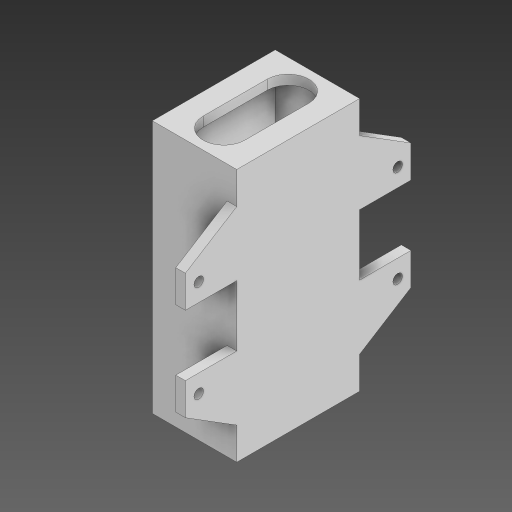
# Autodesk Inventor part: akb_mount
Saved by Autodesk Inventor 2023 (Build 270158000, 158)
## iProperties
Created: 2025-07-15
Part Number: akb_mount
Material: Типовые
Document SubType Name: Modeling
Designer: daa
Density: 1 g/cm^3
Appearance: По умолчанию
Author: daa
Autodesk Inventor part; units mm, degrees
ref_plane "YZ Plane" through (0, 0, 0) normal (1, 0, 0) x (0, 1, 0)
ref_plane "XZ Plane" through (0, 0, 0) normal (0, 1, 0) x (-1, 0, 0)
ref_plane "XY Plane" through (0, 0, 0) normal (0, 0, 1) x (1, 0, 0)
sketch "Эскиз1" plane through (0, 0, 0) normal (0, 1, 0) x (-1, 0, 0)
  line L0 (11, 17) -> (-11, 17)
  line L1 (-11, 17) -> (-11, -17)
  line L2 (-11, -17) -> (11, -17)
  line L3 (11, -17) -> (11, 17)
  line L4 (11, 17) -> (-11, -17) construction
  line L5 (11.65, 17.65) -> (-11.65, 17.65)
  line L6 (-11.65, 17.65) -> (-11.65, -17.65)
  line L7 (-11.65, -17.65) -> (11.65, -17.65)
  line L8 (11.65, -17.65) -> (11.65, 17.65)
  line L9 (11.65, 17.65) -> (-11.65, -17.65) construction
  line L10 (13.15, 19.15) -> (-13.15, 19.15)
  line L11 (-13.15, 19.15) -> (-13.15, -19.15)
  line L12 (-13.15, -19.15) -> (13.15, -19.15)
  line L13 (13.15, -19.15) -> (13.15, 19.15)
  line L14 (13.15, 19.15) -> (-13.15, -19.15) construction
  point P0 (0, 0)
  point P1 (0, 0)
  point P2 (0, 0)
  dimension "d0" = 22
  dimension "d1" = 34
  dimension "d2" = 23.3
  dimension "d3" = 35.3
  dimension "d4" = 26.3
  dimension "d5" = 38.3
  constraints: 30 end point, 6 parallel, 3 horizontal, 3 midpoint, 3 perpendicular, 1 coincident
  measures "d0" distance of L2.end L2.start
  measures "d1" distance of L2.start L0.end
  measures "d2" distance of L7.start L7.end
  measures "d3" distance of L7.end L5.start
  measures "d4" distance of L12.start L12.end
  measures "d5" distance of L10.end L12.start
extrude "Выдавливание1" add sketch "Эскиз1" along normal blind 76 contours L13 L12 L11 L10
sketch "Эскиз2" plane through (0, 76, 0) normal (0, 1, 0) x (1, 0, 0)
  line L0 (11, 17) -> (-11, 17)
  line L1 (-11, 17) -> (-11, -17)
  line L2 (-11, -17) -> (11, -17)
  line L3 (11, -17) -> (11, 17)
  line L4 (11, 17) -> (-11, -17) construction
  line L5 (11.65, 17.65) -> (-11.65, 17.65)
  line L6 (-11.65, 17.65) -> (-11.65, -17.65)
  line L7 (-11.65, -17.65) -> (11.65, -17.65)
  line L8 (11.65, -17.65) -> (11.65, 17.65)
  line L9 (11.65, 17.65) -> (-11.65, -17.65) construction
  line L10 (13.15, 19.15) -> (-13.15, 19.15)
  line L11 (-13.15, 19.15) -> (-13.15, -19.15)
  line L12 (-13.15, -19.15) -> (13.15, -19.15)
  line L13 (13.15, -19.15) -> (13.15, 19.15)
  line L14 (13.15, 19.15) -> (-13.15, -19.15) construction
  point P0 (0, 0)
  point P1 (0, 0)
  point P2 (0, 0)
  dimension "d10" = 22
  dimension "d11" = 34
  dimension "d12" = 23.3
  dimension "d13" = 35.3
  dimension "d14" = 26.3
  dimension "d15" = 38.3
  constraints: 30 end point, 6 parallel, 3 horizontal, 3 midpoint, 3 perpendicular, 1 coincident
  measures "d10" distance of L2.end L2.start
  measures "d11" distance of L2.start L0.end
  measures "d12" distance of L7.start L7.end
  measures "d13" distance of L7.end L5.start
  measures "d14" distance of L12.start L12.end
  measures "d15" distance of L10.end L12.start
extrude "Выдавливание2" add sketch "Эскиз2" along normal blind 3 contours L3 L2 L1 L0 | L8 L7 L6 L5 | L13 L12 L11 L10
sketch "Эскиз3" plane through (0, 79, 0) normal (0, 1, 0) x (1, 0, 0)
  line L0 (0, 10) -> (0, -10) construction
  line L1 (-6.5, 10) -> (-6.5, -10)
  line L2 (6.5, -10) -> (6.5, 10)
  arc A0 (6.5, 10) -> (-6.5, 10) centre (0, 10) ccw
  arc A1 (-6.5, -10) -> (6.5, -10) centre (0, -10) ccw
  line L3 (13.15, -19.15) -> (13.15, 19.15) projected
  line L4 (13.15, 19.15) -> (-13.15, 19.15) projected
  point P0 (0, 0)
  point P1 (13.15, 0)
  dimension "d21" = 20
  dimension "d22" = 13
  dimension "d23" = 6.65
  dimension "d24" = 19.15
  constraints: 8 end point, 4 point on circle, 4 tangent, 2 centre point, 2 midpoint, 1 parallel, 1 vertical
  measures "d21" distance of L0.start L0.end
  measures "d22" diameter of A1
  measures "d23" distance from line of point (13.15, 0) L2
  measures "d24" distance from line of L4 point (0, 0)
extrude "Выдавливание3" cut sketch "Эскиз3" against normal blind 3
sketch "Эскиз4" plane through (13.15, 0, 19.15) normal (1, 0, 0) x (0, 0, -1)
  line L0 (0, 0) -> (0, 79) projected
  line L1 (38.3, 0) -> (38.3, 79) projected
  line L2 (0, 79) -> (38.3, 79)
  line L3 (38.3, 79) -> (38.3, 0)
  line L4 (38.3, 0) -> (0, 0)
  line L5 (0, 0) -> (0, 79)
  circle A0 centre (50.15, 54.6) radius 1.5
  line L6 (50.15, 54.6) -> (-11.85, 54.6)
  line L7 (-11.85, 54.6) -> (-11.85, 24.4)
  line L8 (-11.85, 24.4) -> (50.15, 24.4)
  line L9 (50.15, 24.4) -> (50.15, 54.6)
  circle A1 centre (-11.85, 54.6) radius 1.5
  circle A2 centre (-11.85, 24.4) radius 1.5
  circle A3 centre (50.15, 24.4) radius 1.5
  line L10 (38.3, 79) -> (0, 79) projected
  line L11 (19.15, 79) -> (19.15, 0)
  line L12 (0, 39.5) -> (38.3, 39.5)
  line L13 (38.3, 39.5) -> (0, 39.5)
  circle A4 centre (-11.85, 24.4) radius 1.5
  line L14 (38.3, 49) -> (54.3, 49)
  line L15 (54.3, 49) -> (54.3, 59)
  line L16 (54.3, 59) -> (38.3, 69)
  line L17 (38.3, 30) -> (54.3, 30)
  line L18 (54.3, 30) -> (54.3, 20)
  line L19 (54.3, 20) -> (38.3, 10)
  line L20 (-16, 20) -> (0, 10)
  line L21 (-16, 30) -> (-16, 20)
  line L22 (0, 30) -> (-16, 30)
  line L23 (0, 49) -> (-16, 49)
  line L24 (-16, 49) -> (-16, 59)
  line L25 (-16, 59) -> (0, 69)
  point P0 (54.3, 54)
  point P1 (54.3, 25)
  point P2 (50.15, 30)
  point P3 (50.15, 49)
  point P4 (-11.85, 49)
  point P5 (-11.85, 30)
  dimension "d50" = 3
  dimension "d53" = 62
  dimension "d54" = 30.2
  dimension "d55" = 11.85
  dimension "d56" = 3
  dimension "d57" = 3
  dimension "d61" = 24.4
  dimension "d62" = 30
  dimension "d63" = 10
  dimension "d64" = 10
  dimension "d65" = 4.15
  constraints: 46 end point, 16 symmetric about line, 5 centre point, 5 midpoint, 4 parallel, 3 coincident, 3 horizontal, 2 perpendicular, 2 point on line, 1 vertical, 1 other
  measures "d50" diameter of A0
  measures "d53" distance of L8.end L7.end
  measures "d54" distance of L7.end L6.end
  measures "d55" distance between parallel lines of L0 L7
  measures "d56" diameter of A1
  measures "d57" diameter of A2
  measures "d61" distance between parallel lines of L4 L8
  measures "d62" distance of L14.start L1.end
  measures "d63" distance of L14.end L15.end
  measures "d64" distance of L16.end L1.end
  measures "d65" horizontal distance of point (54.3, 54) L6.start
extrude "Выдавливание5" add sketch "Эскиз4" against normal blind 3 contours L20 L21 L22 L7 A2 L8 L0 | L8 A2 L7 L22 L0 | L1 L8 A3 L9 L17 L18 L19 | L1 L17 L9 A3 L8 | L23 L7 A1 L6 L0 | L23 L24 L25 L0 L6 A1 L7 | L6 A0 L9 L14 L1 | L1 L16 L15 L14 L9 A0 L6
sketch "Эскиз5" plane through (-13.15, 0, -19.15) normal (-1, 0, 0) x (0, 0, 1)
  circle A0 centre (19.15, 5) radius 2.5
  point P0 (19.15, 0)
  dimension "d69" = 5
  constraints: 1 centre point
  measures "d69" diameter of A0
extrude "Выдавливание6" cut sketch "Эскиз5" against normal blind 13.5
equation "\"d2\" = d0 + d6"
equation "\"d3\" = d1 + d6"
equation "\"d4\" = d6 + d0 + d7"
equation "\"d5\" = d6 + d1 + d7"
equation "\"d12\" = d10 + d16"
equation "\"d13\" = d11 + d16"
equation "\"d14\" = d16 + d10 + d17"
equation "\"d15\" = d16 + d11 + d17"
equation "\"d6\" = 1.3"
equation "\"d7\" = 3"
equation "\"d16\" = 1.3"
equation "\"d17\" = 3"
